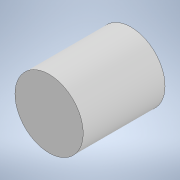
# Autodesk Inventor part: Motors
Saved by Autodesk Inventor 2022 (Build 260153000, 153)
## iProperties
Created: 2021-12-07
Part Number: Motors
Material: Generic
Document SubType Name: Modeling
Designer: Vedic
Density: 1 g/cm^3
Appearance: Default
Author: Vedic
Autodesk Inventor part; units mm, degrees
ref_plane "YZ Plane" through (0, 0, 0) normal (1, 0, 0) x (0, 1, 0)
ref_plane "XZ Plane" through (0, 0, 0) normal (0, 1, 0) x (-1, 0, 0)
ref_plane "XY Plane" through (0, 0, 0) normal (0, 0, 1) x (1, 0, 0)
sketch "Sketch1" plane through (0, 0, 0) normal (0, 0, 1) x (1, 0, 0)
  circle A0 centre (0, 0) radius 63.5
  circle A1 centre (0, 0) radius 35.921 construction
  line L0 (-25.4, 25.4) -> (25.4, 25.4) construction
  line L1 (25.4, 25.4) -> (25.4, -25.4) construction
  line L2 (25.4, -25.4) -> (-25.4, -25.4) construction
  line L3 (-25.4, -25.4) -> (-25.4, 25.4) construction
  circle A2 centre (-25.4, 25.4) radius 3.175
  circle A3 centre (25.4, 25.4) radius 3.175
  circle A4 centre (25.4, -25.4) radius 3.175
  circle A5 centre (-25.4, -25.4) radius 3.175
  dimension "d0" = 127
  dimension "d2" = 6.35
  dimension "d7" = 50.8
  constraints: 8 end point, 6 centre point, 6 coincident, 3 equal radius, 3 point on circle, 2 parallel, 2 perpendicular, 1 horizontal
  measures "d0" diameter of A0
  measures "d2" diameter of A2
  measures "d7" distance of L1.end L2.end
extrude "Extrusion1" add sketch "Sketch1" along normal blind 25.4
sketch "Sketch2" plane through (0, 0, 25.4) normal (0, 0, 1) x (1, 0, 0)
  circle A0 centre (0, 0) radius 63.5
  constraints: 1 centre point, 1 coincident
extrude "Extrusion2" add sketch "Sketch2" along normal blind 127
body "Solid1"
